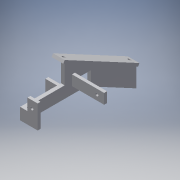
# Autodesk Inventor part: soportefinalfinal
Saved by Autodesk Inventor 2017 (Build 210142000, 142)
## iProperties
Part Number: soportefinalfinal
Material: Genérico
Document SubType Name: Modeling
Designer: Roberto
Density: 1 g/cm^3
Appearance: Valor por defecto
Author: Roberto
Autodesk Inventor part; units mm, degrees
ref_plane "YZ Plane" through (0, 0, 0) normal (1, 0, 0) x (0, 1, 0)
ref_plane "XZ Plane" through (0, 0, 0) normal (0, 1, 0) x (-1, 0, 0)
ref_plane "XY Plane" through (0, 0, 0) normal (0, 0, 1) x (1, 0, 0)
sketch "Boceto1" plane through (0, 0, 0) normal (1, 0, 0) x (0, 1, 0)
  line L0 (0, 0) -> (0, 0.8)
  line L1 (0, 0) -> (2.8, 0)
  line L2 (2.8, 0.8) -> (2.8, 2.3)
  line L3 (0, 0.8) -> (2.8, 0.8)
  line L4 (2.8, 0) -> (3.8, 0)
  line L5 (2.8, 0) -> (4.2826, 0)
  line L6 (7.1, 0) -> (2.8, 2.3)
  line L7 (7.9144, -0.4356) -> (7.1, 0)
  line L8 (7.9144, -0.4356) -> (7.7144, -0.4356)
  line L9 (7.7144, -0.4356) -> (7.7144, -1.8356)
  line L10 (7.7144, -1.8356) -> (6.9, -1.4)
  line L11 (6.9, -1.4) -> (4.2826, 0)
  line L12 (2.8, 2.3) -> (2.8, 0.8)
  line L13 (2.8, 0.8) -> (0, 0.8)
  line L14 (0, 0.8) -> (0, 0)
  line L15 (0, 0) -> (4.2826, 0)
  line L16 (4.2826, 0) -> (7.7144, -1.8356)
  line L17 (7.7144, -1.8356) -> (7.7144, -0.4356)
  line L18 (7.7144, -0.4356) -> (7.9144, -0.4356)
  line L19 (7.9144, -0.4356) -> (2.8, 2.3)
  line L20 (2.8, 2.3) -> (2.8, 0.8)
  dimension "d0" = 0.8
  dimension "d1" = 2.8
  dimension "d2" = 2.3
  dimension "d3" = 1
  dimension "d5" = 4.3
  dimension "d6" = 0.2
  dimension "d7" = 1.4
  constraints: 42 end point, 7 perpendicular, 4 collinear, 3 horizontal, 2 vertical, 1 coincident, 1 parallel
  measures "d0" distance of L0.start L0.end
  measures "d1" distance of L0.start L1.end
  measures "d2" distance of L1.end L2.end
  measures "d3" distance of L1.end L4.end
  measures "d5" distance of L1.end L6.start
  measures "d6" distance of L7.start L8.end
  measures "d7" distance of L8.end L9.end
extrude "Extrusión1" add sketch "Boceto1" against normal blind 0.25
sketch "Boceto2" plane through (0, 0, 0) normal (1, 0, 0) x (0, 0, -1)
  line L0 (0, 0) -> (0, 4.2826) projected
  line L1 (0, 4.2826) -> (1.8356, 7.7144) projected
  line L2 (1.8356, 7.7144) -> (0.4356, 7.7144) projected
  line L3 (0.4356, 7.7144) -> (0.4356, 7.9144) projected
  line L4 (0.4356, 7.9144) -> (-2.3, 2.8) projected
  line L5 (-2.3, 2.8) -> (-0.8, 2.8) projected
  line L6 (-0.8, 2.8) -> (-0.8, 0) projected
  line L7 (-0.8, 0) -> (0, 0) projected
  line L8 (0, 0) -> (0, 2.8)
  line L9 (0, 4.2826) -> (0, 0) projected
  line L10 (0, 3.8) -> (-0.8, 3.8)
  line L11 (-0.8, 3.8) -> (-0.8, 4.6)
  line L12 (-0.8, 4.6) -> (0.1698, 4.6)
  line L13 (0, 3.8) -> (0, 4.2826)
  line L14 (0, 4.2826) -> (0.1698, 4.6)
  line L15 (0, 4.2826) -> (1.8356, 7.7144) projected
  dimension "d10" = 3.8
  dimension "d11" = 0.8
  dimension "d12" = 0.8
  constraints: 12 end point, 3 perpendicular, 2 point on line, 1 collinear
  measures "d10" distance of L0.start L10.start
  measures "d11" distance of L10.start L10.end
  measures "d12" distance of L10.end L11.end
extrude "Extrusión2" cut sketch "Boceto2" against normal blind 0.3 contours L10 L11 L12 L1 L0
sketch "Boceto3" plane through (-0.25, 7.9144, -0.4356) normal (0, 0.4716523, 0.8817846) x (1, 0, 0)
  line L0 (0.25, 0) -> (0, 0) projected
  line L1 (0, -5.8) -> (0, 0) projected
  line L2 (0.25, -5.8) -> (0, -5.8) projected
  line L3 (0, -5.8) -> (0.8, -5.8)
  line L4 (0.8, -5.8) -> (0.8, 0)
  line L5 (0, 0) -> (0.8, 0)
  line L6 (0, 0) -> (0, -5.8)
  line L7 (0, -5.8) -> (0, -5.55)
  circle A0 centre (0.375, -5.425) radius 0.125
  line L8 (0.375, -5.3) -> (0.375, -0.45)
  line L9 (0.375, -5.55) -> (0.4814, -5.7157)
  circle A1 centre (0.375, -0.325) radius 0.125
  point P0 (0.25, -7.1842)
  dimension "d15" = 0.8
  dimension "d16" = 0.8
  dimension "d22" = 4.85
  constraints: 14 end point, 2 centre point, 2 point on circle, 2 vertical, 1 horizontal, 1 perpendicular, 1 point on line
  measures "d15" distance of L1.start L3.end
  measures "d16" distance of L4.end L0.end
  measures "d22" distance of L8.start L8.end
extrude "Extrusión3" add sketch "Boceto3" against normal blind 0.2
sketch "Boceto4" plane through (0, 0, 0) normal (0, -1, 0) x (1, 0, 0)
  line L0 (0, 0.8) -> (0, 0) projected
  line L1 (0, 0) -> (-1.2, 0)
  line L2 (-1.2, 0) -> (-1.2, 1.6)
  line L3 (-1.2, 1.6) -> (-0.5, 1.6)
  line L4 (-0.5, 1.6) -> (-0.5, 0.8)
  line L5 (0, 0.8) -> (-0.5, 0.8)
  line L6 (0, 0.8) -> (0, 0)
  line L7 (-1.2, 0) -> (-1.2, 1.1)
  circle A0 centre (-0.8, 1.1) radius 0.1
  line L8 (-0.6502, 1.1143) -> (-0.6002, 1.1143)
  dimension "d25" = 1.2
  dimension "d26" = 1.6
  dimension "d27" = 0.7
  dimension "d28" = 1.1
  dimension "d58" = 0.05
  constraints: 16 end point, 3 horizontal, 3 perpendicular, 1 centre point, 1 point on line, 1 vertical
  measures "d25" distance of L0.end L1.end
  measures "d26" distance of L1.end L2.end
  measures "d27" distance of L2.end L3.end
  measures "d28" distance of L1.end L7.end
  measures "d58" distance of L8.start L8.end
extrude "Extrusión4" add sketch "Boceto4" against normal blind 0.2
sketch "Boceto5" plane through (-0.25, 0, 0) normal (-1, 0, 0) x (0, 0, 1)
  line L0 (0, 3.8) -> (0, 0.2) projected
  line L1 (0, 0.2) -> (0, 3.5)
  line L2 (0, 3.5) -> (0.5, 3.5)
  line L3 (0.5, 3.5) -> (1.2, 3.5)
  line L4 (1.2, 3.5) -> (1.2, 3.3)
  line L5 (1.2, 3.3) -> (0.5, 3.3)
  line L6 (0.5, 3.3) -> (0.5, 3.5)
  point P0 (0, 0)
  dimension "d33" = 3.3
  dimension "d34" = 0.5
  dimension "d35" = 0.7
  dimension "d36" = 0.2
  dimension "d37" = 0.7
  constraints: 12 end point, 3 perpendicular, 2 point on line
  measures "d33" distance of L0.end L1.end
  measures "d34" distance of L1.end L2.end
  measures "d35" distance of L2.end L3.end
  measures "d36" distance of L3.end L4.end
  measures "d37" distance of L4.end L5.end
extrude "Extrusión5" add sketch "Boceto5" along normal blind 2.2
sketch "Boceto6" plane through (-0.25, 3.5, 1.2) normal (0, 1, 0) x (1, 0, 0)
  line L0 (0, 0.7) -> (-2.2, 0.7) projected
  line L1 (0, 0.7) -> (0, 0.45)
  line L2 (0, 0.4) -> (0, -0.8732) projected
  line L3 (0, 0.45) -> (-1.7, 0.45)
  circle A0 centre (-1.7, 0.35) radius 0.1
  point P0 (0.25, 1.2)
  dimension "d40" = 0.25
  dimension "d41" = 1.7
  constraints: 4 end point, 1 collinear, 1 perpendicular, 1 vertical alignment, 2 other
  measures "d40" distance of L0.start L1.end
  measures "d41" distance of L1.end L3.end
extrude "Extrusión6" cut sketch "Boceto6" against normal blind 2.2
mirror "Simetría1" about plane through (-2.45, 3.4, 0.85) normal (-1, 0, 0) remove original yes
sketch "Boceto9" plane through (-4.9, 7.7144, -1.8356) normal (-1, 0, 0) x (0, 0, 1)
  line L0 (2.6356, -4.9144) -> (3.9088, -4.9144) projected
  line L1 (2.6356, -4.9144) -> (2.6356, -4.9844)
  line L2 (2.6356, -7.5144) -> (2.6356, -4.9144) projected
  line L3 (2.6356, -4.9844) -> (1.8356, -4.9844)
  line L4 (1.8356, -3.9144) -> (1.8356, -7.5144) projected
  line L5 (1.8356, -4.9844) -> (1.8356, -5.1844)
  line L6 (1.8356, -5.1844) -> (2.6356, -5.1844)
  line L7 (2.6356, -4.9844) -> (2.6356, -5.1844)
  point P0 (1.8356, -7.7144)
  dimension "d59" = 0.07
  dimension "d60" = 0.2
  constraints: 10 end point, 4 point on line, 2 perpendicular, 1 collinear
  measures "d59" distance of L0.start L1.end
  measures "d60" distance of L3.end L5.end
extrude "Extrusión9" add sketch "Boceto9" along normal blind 0.8
sketch "Boceto10" plane through (-4.9, 2.73, 0.8) normal (0, 1, 0) x (1, 0, 0)
  line L0 (-0.8, 0) -> (-0.8, 0.8) projected
  line L1 (0, 0.8) -> (0, 0) projected
  circle A0 centre (-0.4, 0.4) radius 0.1
  point P0 (4.9, 0.8)
  dimension "d63" = 0.2
  constraints: 1 centre point
  measures "d63" diameter of A0
extrude "Extrusión10" cut sketch "Boceto10" against normal blind 0.8
